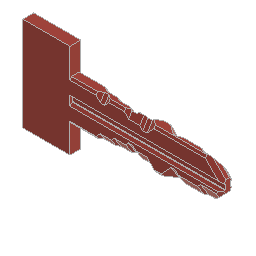
WR (Autodesk Fusion 360 design; units mm, degrees)
Autodesk Fusion 360 part; units mm, degrees
note: some values were not read from the file. Chosen so that the rebuilt part matches the saved one: which face or edge a step refers to. Set by a fixed rule: which sketch regions a step uses.
sketch "blade" plane through (0, 0, 0) normal (1, 0, 0) x (0, 1, 0)
  line L0 (0, 0) -> (1.15, 0) construction
  line L1 (1.15, 0) -> (1.15, 4.3)
  line L2 (1.15, 4.3) -> (-1.15, 4.3)
  line L3 (-1.15, 4.3) -> (-1.15, -4.3)
  line L4 (-1.15, -4.3) -> (1.15, -4.3)
  line L5 (1.15, -4.3) -> (1.15, 0)
  dimension "d61" = 1.15
  dimension "d62" = 4.3
  dimension "d63" = 2.3
  dimension "d64" = 8.6
  constraint coincident L0.start origin
  constraint horizontal L0
  constraint perpendicular L0 L1
  constraint perpendicular L1 L2
  constraint perpendicular L2 L3
  constraint perpendicular L1 L4
  constraint perpendicular L0 L5
  measures "d61" distance of L0.start L0.end
  measures "d62" distance of L0.end L1.end
  measures "d63" distance of L1.end L2.end
  measures "d64" distance of L2.end L3.end
extrude "Extrude1" add sketch "blade" against normal blind 32.35
sketch "centerline" plane through (0, 0, 0) normal (0, 0, 1) x (1, 0, 0)
  line L0 (0, 0) -> (-32.35, 0) construction
  dimension "d67" = 32.35
  constraint coincident L0.start origin
  constraint horizontal L0
  measures "d67" distance of L0.start L0.end
sketch "tip" plane through (0, 0, 0) normal (0, 1, 0) x (1, 0, 0)
  line L0 (0, 0) -> (0, -1.25) construction
  line L1 (0, -1.25) -> (-3.05, -4.3)
  line L2 (0, -1.25) -> (1.25, -1.25) construction
  line L3 (0, 0) -> (1.25, 0) construction
  line L4 (1.25, 0) -> (1.25, -1.25) construction
  line L5 (-3.05, -4.3) -> (0, -4.3)
  line L6 (0, -4.3) -> (0, -1.25)
  line L7 (0, 4.3) -> (0, 1.25)
  line L8 (0, 1.25) -> (-3.05, 4.3)
  line L9 (-3.05, 4.3) -> (0, 4.3)
  dimension "d68" = 1.25
  dimension "d69" = 135
  dimension "d70" = 4.3134
  dimension "d71" = 1.25
  dimension "d72" = 1.25
  constraint coincident L0.start L3.start
  constraint vertical L0
  constraint horizontal L2
  constraint perpendicular L0 L3
  constraint perpendicular L3 L4
  constraint perpendicular L0 L5
  constraint perpendicular L2 L6
  constraint symmetric L0.end L3 L7.end
  constraint symmetric L1.end L3 L8.end
  constraint symmetric L3 L5.end L7.start
  measures "d68" distance of L0.start L0.end
  measures "d69" angle of L1 L2
  measures "d70" distance of L0.end L1.end
  measures "d71" distance of L0.start L3.end
  measures "d72" distance of L3.end L2.end
sketch "warding" plane through (0, 0, 0) normal (1, 0, 0) x (0, 1, 0)
  line L0 (1.15, -4.3) -> (1.15, 4.3)
  line L1 (1.15, 4.3) -> (-1.15, 4.3)
  line L2 (-1.15, 4.3) -> (-1.15, -4.3)
  line L3 (-1.15, -4.3) -> (1.15, -4.3)
  line L4 (0, 0) -> (0.5, 0) construction
  line L5 (0.5, 0) -> (0.5, 0.5)
  line L6 (0.5, 0) -> (0.5, -0.5)
  line L7 (0.5, 0.5) -> (1.15, 0.5)
  line L8 (0.5, -0.5) -> (1.15, -0.5)
  line L9 (0, 0) -> (0, 0.5) construction
  line L10 (-0.5, -0.5) -> (-1.15, -0.5)
  line L11 (-0.5, 0) -> (-0.5, -0.5)
  line L12 (-0.5, 0) -> (-0.5, 0.5)
  line L13 (-0.5, 0.5) -> (-1.15, 0.5)
  dimension "d73" = 0.5
  dimension "d74" = 0.5
  dimension "d75" = 0.5
  dimension "d76" = 0.5
  constraint coincident L4.start L9.start
  constraint perpendicular L0 L4
  constraint perpendicular L4 L5
  constraint perpendicular L4 L6
  constraint coincident L0 L7.end
  constraint perpendicular L0 L7
  constraint coincident L0 L8.end
  constraint perpendicular L0 L8
  constraint perpendicular L4 L9
  constraint symmetric L4.end L9 L11.start
  constraint symmetric L5.end L9 L12.end
  constraint symmetric L6.end L9 L10.start
  constraint symmetric L7.end L9 L13.end
  constraint symmetric L8.end L9 L10.end
  measures "d73" distance of L4.start L4.end
  measures "d74" distance of L4.end L5.end
  measures "d75" distance of L4.end L6.end
  measures "d76" distance of L4.start L9.end
extrude "Extrude2" cut sketch "warding" against normal blind 32.35 contours L0 L5 L6 L7 L8 | L2 L10 L11 L12 L13
chamfer "Chamfer1" distance 0.5 angle 45 4 edges at (-16.175, -1.15, -0.5) (-16.175, 1.15, -0.5) (-16.175, -1.15, 0.5) (-16.175, 1.15, 0.5)
extrude "Extrude3" cut sketch "tip" along normal mid plane 2.3
chamfer "Chamfer2" distance 0.75 angle 45 4 edges at (-1.525, -1.15, 2.775) (-1.525, 1.15, 2.775) (-1.525, -1.15, -2.775) (-1.525, 1.15, -2.775)
ref_plane "WorkPlane1" through (-16.175, 0, 0) normal (0, 0.5373, 0.843391) x (-1, 0, 0)
ref_plane "WorkPlane2" through (-16.175, 0, 0) normal (0, -0.5373, 0.843391) x (-1, 0, 0)
sketch "tr_bl" plane through (0, 0, 0) normal (0, 0.5373, 0.843391) x (-1, 0, 0)
  line L0 (32.35, 0) -> (25.95, 0) construction
  line L1 (25.95, 0) -> (25.45, 0) construction
  line L2 (25.45, 0) -> (25.45, 2.5) construction
  line L3 (25.45, 0) -> (22.45, 0) construction
  line L4 (22.45, 0) -> (22.45, 3) construction
  line L5 (22.45, 0) -> (19.45, 0) construction
  line L6 (19.45, 0) -> (19.45, 2.5) construction
  line L7 (19.45, 0) -> (16.45, 0) construction
  line L8 (16.45, 0) -> (16.45, 2.15) construction
  line L9 (16.45, 0) -> (13.45, 0) construction
  line L10 (13.45, 0) -> (13.45, 3) construction
  line L11 (13.45, 0) -> (10.45, 0) construction
  line L12 (10.45, 0) -> (10.45, 3) construction
  line L13 (10.45, 0) -> (7.45, 0) construction
  line L14 (7.45, 0) -> (7.45, 3) construction
  line L15 (7.45, 0) -> (3.95, 0) construction
  line L16 (3.95, 0) -> (3.95, 3) construction
  line L17 (3.95, 3) -> (0, 3)
  line L18 (0, 3) -> (0, 0) construction
  line L19 (32.35, 0) -> (32.35, 3) construction
  line L20 (32.35, 3) -> (30.45, 3) construction
  line L21 (25.45, 2.5) -> (25.9108, 2.5)
  line L22 (25.45, 0) -> (28.45, 0) construction
  line L23 (28.45, 0) -> (28.45, 3) construction
  line L24 (30.45, 3) -> (28.45, 3)
  line L25 (28.45, 3) -> (26.7768, 3)
  line L26 (26.7768, 3) -> (25.9108, 2.5)
  line L27 (25.45, 2.5) -> (24.9892, 2.5)
  line L28 (22.45, 3) -> (24.1232, 3)
  line L29 (22.45, 3) -> (20.7768, 3)
  line L30 (19.45, 2.5) -> (19.9108, 2.5)
  line L31 (19.45, 2.5) -> (17.517, 2.5)
  line L32 (16.45, 2.15) -> (16.9108, 2.15)
  line L33 (16.45, 2.15) -> (15.9892, 2.15)
  line L34 (13.45, 3) -> (14.517, 3)
  line L35 (13.45, 3) -> (12.9892, 3)
  line L36 (10.45, 3) -> (10.9108, 3)
  line L37 (10.45, 3) -> (9.9892, 3)
  line L38 (7.45, 3) -> (7.9108, 3)
  line L39 (7.45, 3) -> (6.7392, 3)
  line L40 (3.95, 3) -> (4.6608, 3)
  line L41 (4.6608, 3) -> (6.7392, 3)
  line L42 (7.9108, 3) -> (9.9892, 3)
  line L43 (10.9108, 3) -> (12.9892, 3)
  line L44 (14.517, 3) -> (15.9892, 2.15)
  line L45 (16.9108, 2.15) -> (17.517, 2.5)
  line L46 (19.9108, 2.5) -> (20.7768, 3)
  line L47 (24.1232, 3) -> (24.9892, 2.5)
  line L48 (22.45, 0) -> (22.45, -3) construction
  line L49 (10.9108, -3) -> (12.9892, -3)
  line L50 (10.45, -3) -> (9.9892, -3)
  line L51 (25.45, -2.5) -> (25.9108, -2.5)
  line L52 (10.45, 0) -> (10.45, -3) construction
  line L53 (16.9108, -2.15) -> (17.517, -2.5)
  line L54 (25.45, -2.5) -> (24.9892, -2.5)
  line L55 (3.95, -3) -> (0, -3)
  line L56 (7.45, -3) -> (6.7392, -3)
  line L57 (26.7768, -3) -> (25.9108, -2.5)
  line L58 (32.35, -3) -> (30.45, -3) construction
  line L59 (10.45, -3) -> (10.9108, -3)
  line L60 (16.45, 0) -> (16.45, -2.15) construction
  line L61 (22.45, -3) -> (20.7768, -3)
  line L62 (24.1232, -3) -> (24.9892, -2.5)
  line L63 (19.45, 0) -> (19.45, -2.5) construction
  line L64 (28.45, 0) -> (28.45, -3) construction
  line L65 (7.45, -3) -> (7.9108, -3)
  line L66 (13.45, 0) -> (13.45, -3) construction
  line L67 (19.9108, -2.5) -> (20.7768, -3)
  line L68 (19.45, -2.5) -> (17.517, -2.5)
  line L69 (30.45, -3) -> (28.45, -3)
  line L70 (28.45, -3) -> (26.7768, -3)
  line L71 (22.45, -3) -> (24.1232, -3)
  line L72 (16.45, -2.15) -> (16.9108, -2.15)
  line L73 (19.45, -2.5) -> (19.9108, -2.5)
  line L74 (13.45, -3) -> (14.517, -3)
  line L75 (25.45, 0) -> (25.45, -2.5) construction
  line L76 (32.35, 0) -> (32.35, -3) construction
  line L77 (7.45, 0) -> (7.45, -3) construction
  line L78 (13.45, -3) -> (12.9892, -3)
  line L79 (3.95, 0) -> (3.95, -3) construction
  line L80 (3.95, -3) -> (4.6608, -3)
  line L81 (0, -3) -> (0, 0) construction
  line L82 (14.517, -3) -> (15.9892, -2.15)
  line L83 (16.45, -2.15) -> (15.9892, -2.15)
  line L84 (7.9108, -3) -> (9.9892, -3)
  line L85 (4.6608, -3) -> (6.7392, -3)
  point P0 (32.35, 0)
  point P1 (32.35, 0)
  dimension "d86" = 6.4
  dimension "d87" = 0.5
  dimension "d88" = 2.5
  dimension "d89" = 3
  dimension "d90" = 3
  dimension "d91" = 3
  dimension "d92" = 2.5
  dimension "d93" = 3
  dimension "d94" = 2.15
  dimension "d95" = 3
  dimension "d96" = 3
  dimension "d97" = 3
  dimension "d98" = 3
  dimension "d99" = 3
  dimension "d100" = 3
  dimension "d101" = 3.5
  dimension "d102" = 3
  dimension "d103" = 3
  dimension "d104" = 1.9
  dimension "d105" = 0.4608
  dimension "d106" = 3
  dimension "d107" = 3
  dimension "d108" = 1.6732
  dimension "d109" = 0.4608
  dimension "d110" = 1.6732
  dimension "d111" = 1.6732
  dimension "d112" = 0.4608
  dimension "d113" = 1.933
  dimension "d114" = 0.4608
  dimension "d115" = 0.4608
  dimension "d116" = 1.067
  dimension "d117" = 0.4608
  dimension "d118" = 0.4608
  dimension "d119" = 0.4608
  dimension "d120" = 0.4608
  dimension "d121" = 0.7108
  dimension "d122" = 0.7108
  constraint coincident P0 L0.start
  constraint coincident P1 P0
  constraint horizontal L0
  constraint parallel L0 L1
  constraint perpendicular L1 L2
  constraint perpendicular L2 L3
  constraint perpendicular L3 L4
  constraint perpendicular L4 L5
  constraint perpendicular L5 L6
  constraint perpendicular L6 L7
  constraint perpendicular L7 L8
  constraint perpendicular L8 L9
  constraint perpendicular L9 L10
  constraint perpendicular L10 L11
  constraint perpendicular L11 L12
  constraint perpendicular L12 L13
  constraint perpendicular L13 L14
  constraint perpendicular L14 L15
  constraint perpendicular L15 L16
  constraint perpendicular L16 L17
  constraint coincident L18.end L81.end
  constraint perpendicular L17 L18
  constraint perpendicular L0 L19
  constraint perpendicular L19 L20
  constraint perpendicular L2 L21
  constraint perpendicular L2 L22
  constraint perpendicular L22 L23
  constraint perpendicular L23 L25
  constraint perpendicular L2 L27
  constraint perpendicular L4 L28
  constraint perpendicular L4 L29
  constraint perpendicular L6 L30
  constraint perpendicular L6 L31
  constraint perpendicular L8 L32
  constraint perpendicular L8 L33
  constraint perpendicular L10 L34
  constraint perpendicular L10 L35
  constraint perpendicular L12 L36
  constraint perpendicular L12 L37
  constraint perpendicular L14 L38
  constraint perpendicular L14 L39
  constraint perpendicular L16 L40
  constraint symmetric L1.end L7 L2.start
  constraint symmetric L2.end L7 L51.start
  constraint symmetric L3.end L7 L4.start
  constraint symmetric L4.end L7 L48.end
  constraint symmetric L5.end L7 L6.start
  constraint symmetric L6.end L7 L63.end
  constraint symmetric L8.start L7 L9.start
  constraint symmetric L7 L8.end L60.end
  constraint symmetric L7 L9.end L10.start
  constraint symmetric L7 L10.end L66.end
  constraint symmetric L7 L11.end L12.start
  constraint symmetric L7 L12.end L50.start
  constraint symmetric L7 L13.end L14.start
  constraint symmetric L7 L14.end L56.start
  constraint symmetric L7 L15.end L16.start
  constraint symmetric L7 L16.end L55.start
  constraint symmetric L7 L17.end L55.end
  constraint symmetric L7 L18.end L81.end
  constraint symmetric L7 P1 P0
  constraint symmetric L7 L19.end L58.start
  constraint symmetric L7 L20.end L58.end
  constraint symmetric L7 L21.end L51.end
  constraint symmetric L7 L22.end L23.start
  constraint symmetric L7 L23.end L64.end
  constraint symmetric L7 L25.end L57.start
  constraint symmetric L7 L27.end L54.end
  constraint symmetric L7 L28.end L62.start
  constraint symmetric L7 L29.end L61.end
  constraint symmetric L7 L30.end L67.start
  constraint symmetric L7 L31.end L53.end
  constraint symmetric L7 L32.end L53.start
  constraint symmetric L7 L33.end L82.end
  constraint symmetric L7 L34.end L74.end
  constraint symmetric L7 L35.end L49.end
  constraint symmetric L7 L36.end L49.start
  constraint symmetric L7 L37.end L50.end
  constraint symmetric L7 L38.end L65.end
  constraint symmetric L7 L39.end L56.end
  constraint symmetric L7 L40.end L80.end
  measures "d86" distance of P1 L0.end
  measures "d87" distance of L0.end L1.end
  measures "d88" distance of L1.end L2.end
  measures "d89" distance of L1.end L3.end
  measures "d90" distance of L3.end L4.end
  measures "d91" distance of L3.end L5.end
  measures "d92" distance of L5.end L6.end
  measures "d93" distance of L5.end L7.end
  measures "d94" distance of L7.end L8.end
  measures "d95" distance of L7.end L9.end
  measures "d96" distance of L9.end L10.end
  measures "d97" distance of L9.end L11.end
  measures "d98" distance of L11.end L12.end
  measures "d99" distance of L11.end L13.end
  measures "d100" distance of L13.end L14.end
  measures "d101" distance of L13.end L15.end
  measures "d102" distance of L15.end L16.end
  measures "d103" distance of P1 L19.end
  measures "d104" distance of L19.end L20.end
  measures "d105" distance of L2.end L21.end
  measures "d106" distance of L1.end L22.end
  measures "d107" distance of L22.end L23.end
  measures "d108" distance of L23.end L25.end
  measures "d109" distance of L2.end L27.end
  measures "d110" distance of L4.end L28.end
  measures "d111" distance of L4.end L29.end
  measures "d112" distance of L6.end L30.end
  measures "d113" distance of L6.end L31.end
  measures "d114" distance of L8.end L32.end
  measures "d115" distance of L8.end L33.end
  measures "d116" distance of L10.end L34.end
  measures "d117" distance of L10.end L35.end
  measures "d118" distance of L12.end L36.end
  measures "d119" distance of L12.end L37.end
  measures "d120" distance of L14.end L38.end
  measures "d121" distance of L14.end L39.end
  measures "d122" distance of L16.end L40.end
sketch "tr_bl cutters" plane through (0, 0, 0) normal (1, 0, 0) x (0, 1, 0)
  line L0 (0, 0) -> (-2.5302, 1.6119) construction
  line L1 (0, 0) -> (-3.5571, 0) construction
  line L2 (-2.5302, 1.6119) -> (-0.1123, 5.4072)
  line L3 (-2.5302, 1.6119) -> (-4.948, -2.1834)
  line L4 (-0.1123, 5.4072) -> (-4.948, 5.4072)
  line L5 (-4.948, 5.4072) -> (-4.948, -2.1834)
  line L6 (0, 0) -> (2.5302, -1.6119) construction
  line L7 (2.5302, -1.6119) -> (0.1123, -5.4072)
  line L8 (2.5302, -1.6119) -> (4.948, 2.1834)
  line L9 (0.1123, -5.4072) -> (4.948, -5.4072)
  line L10 (4.948, -5.4072) -> (4.948, 2.1834)
  dimension "d123" = 147.5
  dimension "d124" = 3
  dimension "d126" = 4.5
  dimension "d127" = 4.5
  dimension "d128" = 3
  dimension "d129" = 4.5
  dimension "d130" = 4.5
  constraint horizontal L1
  constraint coincident L0.start L1.start
  constraint perpendicular L0 L2
  constraint perpendicular L0 L3
  constraint horizontal L4
  constraint perpendicular L4 L5
  constraint coincident L1.end L3
  constraint parallel L0 L6
  constraint perpendicular L6 L7
  constraint perpendicular L6 L8
  constraint horizontal L9
  constraint perpendicular L9 L10
  measures "d123" angle of L0 L1
  measures "d124" distance of L0.start L0.end
  measures "d126" distance of L0.end L2.end
  measures "d127" distance of L0.end L3.end
  measures "d128" distance of L0.start L6.end
  measures "d129" distance of L6.end L7.end
  measures "d130" distance of L6.end L8.end
sketch "tl_br" plane through (0, 0, 0) normal (0, -0.5373, 0.843391) x (-1, 0, 0)
  line L0 (32.35, 0) -> (25.95, 0) construction
  line L1 (25.95, 0) -> (25.45, 0) construction
  line L2 (25.45, 0) -> (25.45, -2.5) construction
  line L3 (25.45, 0) -> (22.45, 0) construction
  line L4 (22.45, 0) -> (22.45, -2.15) construction
  line L5 (22.45, 0) -> (19.45, 0) construction
  line L6 (19.45, 0) -> (19.45, -1.8) construction
  line L7 (19.45, 0) -> (16.45, 0) construction
  line L8 (16.45, 0) -> (16.45, -2.15) construction
  line L9 (16.45, 0) -> (13.45, 0) construction
  line L10 (13.45, 0) -> (13.45, -3) construction
  line L11 (13.45, 0) -> (10.45, 0) construction
  line L12 (10.45, 0) -> (10.45, -1.8) construction
  line L13 (10.45, 0) -> (7.45, 0) construction
  line L14 (7.45, 0) -> (7.45, -2.15) construction
  line L15 (7.45, 0) -> (3.95, 0) construction
  line L16 (3.95, 0) -> (3.95, -1.8) construction
  line L17 (3.95, -1.8) -> (0, -1.8)
  line L18 (0, -1.8) -> (0, 0) construction
  line L19 (32.35, 0) -> (32.35, -3) construction
  line L20 (32.35, -3) -> (30.45, -3) construction
  line L21 (25.45, 0) -> (28.45, 0) construction
  line L22 (28.45, 0) -> (28.45, -3) construction
  line L23 (28.45, -3) -> (30.45, -3)
  line L24 (25.45, -2.5) -> (25.9108, -2.5)
  line L25 (28.45, -3) -> (26.7768, -3)
  line L26 (26.7768, -3) -> (25.9108, -2.5)
  line L27 (25.45, -2.5) -> (23.517, -2.5)
  line L28 (22.45, -2.15) -> (22.9108, -2.15)
  line L29 (22.45, -2.15) -> (20.517, -2.15)
  line L30 (19.45, -1.8) -> (19.9108, -1.8)
  line L31 (19.45, -1.8) -> (18.9892, -1.8)
  line L32 (16.45, -2.15) -> (18.383, -2.15)
  line L33 (16.45, -2.15) -> (15.9892, -2.15)
  line L34 (13.45, -3) -> (14.517, -3)
  line L35 (13.45, -3) -> (12.9892, -3)
  line L36 (10.45, -1.8) -> (10.9108, -1.8)
  line L37 (10.45, -1.8) -> (9.9892, -1.8)
  line L38 (7.45, -2.15) -> (9.383, -2.15)
  line L39 (7.45, -2.15) -> (5.267, -2.15)
  line L40 (3.95, -1.8) -> (4.6608, -1.8)
  line L41 (4.6608, -1.8) -> (5.267, -2.15)
  line L42 (9.383, -2.15) -> (9.9892, -1.8)
  line L43 (10.9108, -1.8) -> (12.9892, -3)
  line L44 (14.517, -3) -> (15.9892, -2.15)
  line L45 (18.383, -2.15) -> (18.9892, -1.8)
  line L46 (19.9108, -1.8) -> (20.517, -2.15)
  line L47 (22.9108, -2.15) -> (23.517, -2.5)
  line L48 (22.45, 0) -> (22.45, 2.15) construction
  line L49 (19.45, 1.8) -> (18.9892, 1.8)
  line L50 (22.45, 2.15) -> (20.517, 2.15)
  line L51 (22.45, 2.15) -> (22.9108, 2.15)
  line L52 (19.9108, 1.8) -> (20.517, 2.15)
  line L53 (25.45, 2.5) -> (23.517, 2.5)
  line L54 (7.45, 2.15) -> (9.383, 2.15)
  line L55 (7.45, 0) -> (7.45, 2.15) construction
  line L56 (3.95, 0) -> (3.95, 1.8) construction
  line L57 (28.45, 3) -> (30.45, 3)
  line L58 (28.45, 0) -> (28.45, 3) construction
  line L59 (25.45, 0) -> (25.45, 2.5) construction
  line L60 (0, 1.8) -> (0, 0) construction
  line L61 (28.45, 3) -> (26.7768, 3)
  line L62 (32.35, 3) -> (30.45, 3) construction
  line L63 (25.45, 2.5) -> (25.9108, 2.5)
  line L64 (22.9108, 2.15) -> (23.517, 2.5)
  line L65 (9.383, 2.15) -> (9.9892, 1.8)
  line L66 (18.383, 2.15) -> (18.9892, 1.8)
  line L67 (19.45, 1.8) -> (19.9108, 1.8)
  line L68 (10.45, 1.8) -> (10.9108, 1.8)
  line L69 (16.45, 2.15) -> (18.383, 2.15)
  line L70 (10.45, 1.8) -> (9.9892, 1.8)
  line L71 (14.517, 3) -> (15.9892, 2.15)
  line L72 (10.9108, 1.8) -> (12.9892, 3)
  line L73 (13.45, 3) -> (14.517, 3)
  line L74 (13.45, 0) -> (13.45, 3) construction
  line L75 (13.45, 3) -> (12.9892, 3)
  line L76 (7.45, 2.15) -> (5.267, 2.15)
  line L77 (10.45, 0) -> (10.45, 1.8) construction
  line L78 (19.45, 0) -> (19.45, 1.8) construction
  line L79 (26.7768, 3) -> (25.9108, 2.5)
  line L80 (32.35, 0) -> (32.35, 3) construction
  line L81 (16.45, 2.15) -> (15.9892, 2.15)
  line L82 (3.95, 1.8) -> (4.6608, 1.8)
  line L83 (3.95, 1.8) -> (0, 1.8)
  line L84 (16.45, 0) -> (16.45, 2.15) construction
  line L85 (4.6608, 1.8) -> (5.267, 2.15)
  point P0 (32.35, 0)
  point P1 (32.35, 0)
  dimension "d131" = 6.4
  dimension "d132" = 0.5
  dimension "d133" = 2.5
  dimension "d134" = 3
  dimension "d135" = 2.15
  dimension "d136" = 3
  dimension "d137" = 1.8
  dimension "d138" = 3
  dimension "d139" = 2.15
  dimension "d140" = 3
  dimension "d141" = 3
  dimension "d142" = 3
  dimension "d143" = 1.8
  dimension "d144" = 3
  dimension "d145" = 2.15
  dimension "d146" = 3.5
  dimension "d147" = 1.8
  dimension "d148" = 3
  dimension "d149" = 1.9
  dimension "d150" = 3
  dimension "d151" = 3
  dimension "d152" = 0.4608
  dimension "d153" = 1.6732
  dimension "d154" = 1.933
  dimension "d155" = 0.4608
  dimension "d156" = 1.933
  dimension "d157" = 0.4608
  dimension "d158" = 0.4608
  dimension "d159" = 1.933
  dimension "d160" = 0.4608
  dimension "d161" = 1.067
  dimension "d162" = 0.4608
  dimension "d163" = 0.4608
  dimension "d164" = 0.4608
  dimension "d165" = 1.933
  dimension "d166" = 2.183
  dimension "d167" = 0.7108
  constraint coincident P0 L0.start
  constraint horizontal L0
  constraint parallel L0 L1
  constraint perpendicular L1 L2
  constraint perpendicular L2 L3
  constraint perpendicular L3 L4
  constraint perpendicular L4 L5
  constraint perpendicular L5 L6
  constraint perpendicular L6 L7
  constraint perpendicular L7 L8
  constraint perpendicular L8 L9
  constraint perpendicular L9 L10
  constraint perpendicular L10 L11
  constraint perpendicular L11 L12
  constraint perpendicular L12 L13
  constraint perpendicular L13 L14
  constraint perpendicular L14 L15
  constraint perpendicular L15 L16
  constraint perpendicular L16 L17
  constraint coincident L18.end L60.end
  constraint perpendicular L17 L18
  constraint coincident P1 P0
  constraint perpendicular L0 L19
  constraint perpendicular L19 L20
  constraint perpendicular L2 L21
  constraint perpendicular L21 L22
  constraint perpendicular L2 L24
  constraint perpendicular L22 L25
  constraint perpendicular L2 L27
  constraint perpendicular L4 L28
  constraint perpendicular L4 L29
  constraint perpendicular L6 L30
  constraint perpendicular L6 L31
  constraint perpendicular L8 L32
  constraint perpendicular L8 L33
  constraint perpendicular L10 L34
  constraint perpendicular L10 L35
  constraint perpendicular L12 L36
  constraint perpendicular L12 L37
  constraint perpendicular L14 L38
  constraint perpendicular L14 L39
  constraint perpendicular L16 L40
  constraint symmetric L1.end L7 L2.start
  constraint symmetric L2.end L7 L53.start
  constraint symmetric L3.end L7 L4.start
  constraint symmetric L4.end L7 L48.end
  constraint symmetric L5.end L7 L6.start
  constraint symmetric L6.end L7 L49.start
  constraint symmetric L8.start L7 L9.start
  constraint symmetric L7 L8.end L69.start
  constraint symmetric L7 L9.end L10.start
  constraint symmetric L7 L10.end L73.start
  constraint symmetric L7 L11.end L12.start
  constraint symmetric L7 L12.end L68.start
  constraint symmetric L7 L13.end L14.start
  constraint symmetric L7 L14.end L54.start
  constraint symmetric L7 L15.end L16.start
  constraint symmetric L7 L16.end L56.end
  constraint symmetric L7 L17.end L60.start
  constraint symmetric L7 L18.end L60.end
  constraint symmetric L7 P1 P0
  constraint symmetric L7 L19.end L62.start
  constraint symmetric L7 L20.end L57.end
  constraint symmetric L7 L21.end L22.start
  constraint symmetric L7 L22.end L57.start
  constraint symmetric L7 L24.end L63.end
  constraint symmetric L7 L25.end L61.end
  constraint symmetric L7 L27.end L53.end
  constraint symmetric L7 L28.end L51.end
  constraint symmetric L7 L29.end L50.end
  constraint symmetric L7 L30.end L52.start
  constraint symmetric L7 L31.end L49.end
  constraint symmetric L7 L32.end L66.start
  constraint symmetric L7 L33.end L71.end
  constraint symmetric L7 L34.end L71.start
  constraint symmetric L7 L35.end L72.end
  constraint symmetric L7 L36.end L68.end
  constraint symmetric L7 L37.end L65.end
  constraint symmetric L7 L38.end L54.end
  constraint symmetric L7 L39.end L76.end
  constraint symmetric L7 L40.end L82.end
  measures "d131" distance of P1 L0.end
  measures "d132" distance of L0.end L1.end
  measures "d133" distance of L1.end L2.end
  measures "d134" distance of L1.end L3.end
  measures "d135" distance of L3.end L4.end
  measures "d136" distance of L3.end L5.end
  measures "d137" distance of L5.end L6.end
  measures "d138" distance of L5.end L7.end
  measures "d139" distance of L7.end L8.end
  measures "d140" distance of L7.end L9.end
  measures "d141" distance of L9.end L10.end
  measures "d142" distance of L9.end L11.end
  measures "d143" distance of L11.end L12.end
  measures "d144" distance of L11.end L13.end
  measures "d145" distance of L13.end L14.end
  measures "d146" distance of L13.end L15.end
  measures "d147" distance of L15.end L16.end
  measures "d148" distance of P1 L19.end
  measures "d149" distance of L19.end L20.end
  measures "d150" distance of L1.end L21.end
  measures "d151" distance of L21.end L22.end
  measures "d152" distance of L2.end L24.end
  measures "d153" distance of L22.end L25.end
  measures "d154" distance of L2.end L27.end
  measures "d155" distance of L4.end L28.end
  measures "d156" distance of L4.end L29.end
  measures "d157" distance of L6.end L30.end
  measures "d158" distance of L6.end L31.end
  measures "d159" distance of L8.end L32.end
  measures "d160" distance of L8.end L33.end
  measures "d161" distance of L10.end L34.end
  measures "d162" distance of L10.end L35.end
  measures "d163" distance of L12.end L36.end
  measures "d164" distance of L12.end L37.end
  measures "d165" distance of L14.end L38.end
  measures "d166" distance of L14.end L39.end
  measures "d167" distance of L16.end L40.end
sketch "tl_br cutters" plane through (0, 0, 0) normal (1, 0, 0) x (0, 1, 0)
  line L0 (0, 0) -> (1.5181, 0.9671) construction
  line L1 (0, 0) -> (2.1342, 0) construction
  line L2 (1.5181, 0.9671) -> (-0.8997, 4.7624)
  line L3 (1.5181, 0.9671) -> (3.936, -2.8281)
  line L4 (-0.8997, 4.7624) -> (3.936, 4.7624)
  line L5 (3.936, 4.7624) -> (3.936, -2.8281)
  line L6 (0, 0) -> (-1.5181, -0.9671) construction
  line L7 (-1.5181, -0.9671) -> (-3.936, 2.8281)
  line L8 (-1.5181, -0.9671) -> (0.8997, -4.7624)
  line L9 (0.8997, -4.7624) -> (-3.936, -4.7624)
  line L10 (-3.936, -4.7624) -> (-3.936, 2.8281)
  dimension "d168" = 1.8
  dimension "d169" = 32.5
  dimension "d170" = 4.5
  dimension "d171" = 4.5
  dimension "d172" = 1.8
  dimension "d173" = 4.5
  dimension "d174" = 4.5
  constraint horizontal L1
  constraint coincident L0.start L1.start
  constraint perpendicular L0 L2
  constraint perpendicular L0 L3
  constraint coincident L1.end L3
  constraint horizontal L4
  constraint perpendicular L4 L5
  constraint parallel L0 L6
  constraint perpendicular L6 L7
  constraint perpendicular L6 L8
  constraint horizontal L9
  constraint perpendicular L9 L10
  measures "d168" distance of L0.start L0.end
  measures "d169" angle of L0 L1
  measures "d170" distance of L0.end L2.end
  measures "d171" distance of L0.end L3.end
  measures "d172" distance of L0.start L6.end
  measures "d173" distance of L6.end L7.end
  measures "d174" distance of L6.end L8.end
sweep "Sweep1" cut profiles "tr_bl cutters" path "tr_bl" along L17 L40 L41 L39 L38 L42 L37 L36 L43 L35 L34 L44 L33 L32 L45 L31 L30 L46 L29 L28 L47 L27 L21 L26 L25 L24 section 1 contours L2 L3 L4 L5
sweep "Sweep2" cut profiles "tr_bl cutters" path "tr_bl" along L69 L70 L57 L51 L54 L62 L71 L61 L67 L73 L68 L53 L72 L83 L82 L74 L78 L49 L59 L50 L84 L65 L56 L85 L80 L55 section 1 contours L7 L8 L9 L10
sweep "Sweep3" cut profiles "tl_br cutters" path "tl_br" along L23 L25 L26 L24 L27 L47 L28 L29 L46 L30 L31 L45 L32 L33 L44 L34 L35 L43 L36 L37 L42 L38 L39 L41 L40 L17 section 1 contours L2 L3 L4 L5
sweep "Sweep4" cut profiles "tl_br cutters" path "tl_br" along L83 L82 L85 L76 L54 L65 L70 L68 L72 L75 L73 L71 L81 L69 L66 L49 L67 L52 L50 L51 L64 L53 L63 L79 L61 L57 section 1 contours L7 L8 L9 L10
sketch "Sketch9" plane through (-32.35, 0, 0) normal (-1, 0, 0) x (0, -1, 0)
  line L0 (-1.15, 1) -> (-0.65, 0.5)
  line L1 (-0.65, 0.5) -> (-0.5, 0.5)
  line L2 (-0.5, 0.5) -> (-0.5, -0.5)
  line L3 (-0.5, -0.5) -> (-0.65, -0.5)
  line L4 (-0.65, -0.5) -> (-1.15, -1)
  line L5 (-1.15, -1) -> (-1.15, -4.3)
  line L6 (-1.15, -4.3) -> (1.15, -4.3)
  line L7 (1.15, -4.3) -> (1.15, -1)
  line L8 (1.15, -1) -> (0.65, -0.5)
  line L9 (0.65, -0.5) -> (0.5, -0.5)
  line L10 (0.5, -0.5) -> (0.5, 0.5)
  line L11 (0.5, 0.5) -> (0.65, 0.5)
  line L12 (0.65, 0.5) -> (1.15, 1)
  line L13 (1.15, 1) -> (1.15, 4.3)
  line L14 (1.15, 4.3) -> (-1.15, 4.3)
  line L15 (-1.15, 4.3) -> (-1.15, 1)
  line L16 (1.15, 10) -> (-1.15, 10)
  line L17 (-1.15, 10) -> (-1.15, -10)
  line L18 (-1.15, -10) -> (1.15, -10)
  line L19 (1.15, -10) -> (1.15, 10)
  line L20 (1.15, 10) -> (-1.15, -10) construction
  line L21 (-1.15, 10) -> (1.15, -10) construction
  dimension "d199" = 2.3
  dimension "d200" = 20
  constraint horizontal L16
  constraint perpendicular L16 L17
  constraint parallel L16 L18
  constraint parallel L17 L19
  constraint coincident L20 origin
  constraint coincident L21 origin
  measures "d199" distance of L17.end L18.end
  measures "d200" distance of L16.end L17.end
extrude "Extrude4" add sketch "Sketch9" along normal blind 10
extrude "Extrude5" cut 4 faces at (-30.45, 1.0392, 4.1261) (-30.45, -1.0392, 4.1261) (-30.45, 1.0392, -4.1261) (-30.45, -1.0392, -4.1261) along direction (-1, 0, 0) blind 1.9
equation "tr_bl1 = 1"
equation "trbl1 = ( -0.025 * tr_bl1 ^ 3 + 0.15 * tr_bl1 ^ 2 - 0.625 * tr_bl1 + 3 )"
equation "tr_bl2 = 0"
equation "trbl2 = ( -0.025 * tr_bl2 ^ 3 + 0.15 * tr_bl2 ^ 2 - 0.625 * tr_bl2 + 3 )"
equation "tr_bl3 = 1"
equation "trbl3 = ( -0.025 * tr_bl3 ^ 3 + 0.15 * tr_bl3 ^ 2 - 0.625 * tr_bl3 + 3 )"
equation "tr_bl4 = 2"
equation "trbl4 = ( -0.025 * tr_bl4 ^ 3 + 0.15 * tr_bl4 ^ 2 - 0.625 * tr_bl4 + 3 )"
equation "tr_bl5 = 0"
equation "trbl5 = ( -0.025 * tr_bl5 ^ 3 + 0.15 * tr_bl5 ^ 2 - 0.625 * tr_bl5 + 3 )"
equation "tr_bl6 = 0"
equation "trbl6 = ( -0.025 * tr_bl6 ^ 3 + 0.15 * tr_bl6 ^ 2 - 0.625 * tr_bl6 + 3 )"
equation "tr_bl7 = 0"
equation "trbl7 = ( -0.025 * tr_bl7 ^ 3 + 0.15 * tr_bl7 ^ 2 - 0.625 * tr_bl7 + 3 )"
equation "tr_bl8 = 0"
equation "trbl8 = ( -0.025 * tr_bl8 ^ 3 + 0.15 * tr_bl8 ^ 2 - 0.625 * tr_bl8 + 3 )"
equation "tr1_right = if(( trbl1 > trbl2 ) and ( ( abs(trbl1 - trbl2) ) <> 1.2 ) and ( ( trbl1 - trbl2 ) <> 0 ); 3 mm - ( ( 3 mm - ( ( ( 2.4 * cos(30 deg) ) * 1 mm ) ) ) / 2 ) - ( ( ( trbl1 - trbl2 ) * 2 * cos(30 deg) ) * 1 mm ); if(( trbl1 < trbl2 ) and ( ( abs(trbl1 - trbl2) ) <> 1.2 ) and ( ( trbl1 - trbl2 ) <> 0 ); ( ( 3 - ( 2.40 * cos(30 deg) ) ) / 2 ) * 1 mm; if(( ( abs(trbl1 - trbl2) ) <> 1.2 ) or ( ( trbl1 - trbl2 ) <> 0 ); ( ( 3 - ( 2.40 * cos(30 deg) ) ) / 2 ) * 1 mm; 1 mm)))"
equation "tr2_left = if(( trbl1 < trbl2 ) and ( ( abs(trbl1 - trbl2) ) <> 1.2 ) and ( ( trbl1 - trbl2 ) <> 0 ); 3 mm - ( ( 3 mm - ( ( ( 2.4 * cos(30 deg) ) * 1 mm ) ) ) / 2 ) - ( ( ( trbl2 - trbl1 ) * 2 * cos(30 deg) ) * 1 mm ); if(( trbl1 > trbl2 ) and ( ( abs(trbl1 - trbl2) ) <> 1.2 ) and ( ( trbl1 - trbl2 ) <> 0 ); ( ( 3 - ( 2.40 * cos(30 deg) ) ) / 2 ) * 1 mm; if(( ( abs(trbl2 - trbl1) ) <> 1.2 ) or ( ( trbl1 - trbl2 ) <> 0 ); ( ( 3 - ( 2.40 * cos(30 deg) ) ) / 2 ) * 1 mm; 1 mm)))"
equation "tr2_right = if(( trbl2 > trbl3 ) and ( ( abs(trbl2 - trbl3) ) <> 1.2 ) and ( ( trbl2 - trbl3 ) <> 0 ); 3 mm - ( ( 3 mm - ( ( ( 2.4 * cos(30 deg) ) * 1 mm ) ) ) / 2 ) - ( ( ( trbl2 - trbl3 ) * 2 * cos(30 deg) ) * 1 mm ); if(( trbl2 < trbl3 ) and ( ( abs(trbl2 - trbl3) ) <> 1.2 ) and ( ( trbl2 - trbl3 ) <> 0 ); ( ( 3 - ( 2.40 * cos(30 deg) ) ) / 2 ) * 1 mm; if(( ( abs(trbl2 - trbl3) ) <> 1.2 ) or ( ( trbl2 - trbl3 ) <> 0 ); ( ( 3 - ( 2.40 * cos(30 deg) ) ) / 2 ) * 1 mm; 1 mm)))"
equation "tr3_left = if(( trbl2 < trbl3 ) and ( ( abs(trbl2 - trbl3) ) <> 1.2 ) and ( ( trbl2 - trbl3 ) <> 0 ); 3 mm - ( ( 3 mm - ( ( ( 2.4 * cos(30 deg) ) * 1 mm ) ) ) / 2 ) - ( ( ( trbl3 - trbl2 ) * 2 * cos(30 deg) ) * 1 mm ); if(( trbl2 > trbl3 ) and ( ( abs(trbl2 - trbl3) ) <> 1.2 ) and ( ( trbl2 - trbl3 ) <> 0 ); ( ( 3 - ( 2.40 * cos(30 deg) ) ) / 2 ) * 1 mm; if(( ( abs(trbl3 - trbl2) ) <> 1.2 ) or ( ( trbl2 - trbl3 ) <> 0 ); ( ( 3 - ( 2.40 * cos(30 deg) ) ) / 2 ) * 1 mm; 1 mm)))"
equation "tr3_right = if(( trbl3 > trbl4 ) and ( ( abs(trbl3 - trbl4) ) <> 1.2 ) and ( ( trbl3 - trbl4 ) <> 0 ); 3 mm - ( ( 3 mm - ( ( ( 2.4 * cos(30 deg) ) * 1 mm ) ) ) / 2 ) - ( ( ( trbl3 - trbl4 ) * 2 * cos(30 deg) ) * 1 mm ); if(( trbl3 < trbl4 ) and ( ( abs(trbl3 - trbl4) ) <> 1.2 ) and ( ( trbl3 - trbl4 ) <> 0 ); ( ( 3 - ( 2.40 * cos(30 deg) ) ) / 2 ) * 1 mm; if(( ( abs(trbl3 - trbl4) ) <> 1.2 ) or ( ( trbl3 - trbl4 ) <> 0 ); ( ( 3 - ( 2.40 * cos(30 deg) ) ) / 2 ) * 1 mm; 1 mm)))"
equation "tr4_left = if(( trbl3 < trbl4 ) and ( ( abs(trbl3 - trbl4) ) <> 1.2 ) and ( ( trbl3 - trbl4 ) <> 0 ); 3 mm - ( ( 3 mm - ( ( ( 2.4 * cos(30 deg) ) * 1 mm ) ) ) / 2 ) - ( ( ( trbl4 - trbl3 ) * 2 * cos(30 deg) ) * 1 mm ); if(( trbl3 > trbl4 ) and ( ( abs(trbl3 - trbl4) ) <> 1.2 ) and ( ( trbl3 - trbl4 ) <> 0 ); ( ( 3 - ( 2.40 * cos(30 deg) ) ) / 2 ) * 1 mm; if(( ( abs(trbl4 - trbl3) ) <> 1.2 ) or ( ( trbl3 - trbl4 ) <> 0 ); ( ( 3 - ( 2.40 * cos(30 deg) ) ) / 2 ) * 1 mm; 1 mm)))"
equation "tr4_right = if(( trbl4 > trbl5 ) and ( ( abs(trbl4 - trbl5) ) <> 1.2 ) and ( ( trbl4 - trbl5 ) <> 0 ); 3 mm - ( ( 3 mm - ( ( ( 2.4 * cos(30 deg) ) * 1 mm ) ) ) / 2 ) - ( ( ( trbl4 - trbl5 ) * 2 * cos(30 deg) ) * 1 mm ); if(( trbl4 < trbl5 ) and ( ( abs(trbl4 - trbl5) ) <> 1.2 ) and ( ( trbl4 - trbl5 ) <> 0 ); ( ( 3 - ( 2.40 * cos(30 deg) ) ) / 2 ) * 1 mm; if(( ( abs(trbl4 - trbl5) ) <> 1.2 ) or ( ( trbl4 - trbl5 ) <> 0 ); ( ( 3 - ( 2.40 * cos(30 deg) ) ) / 2 ) * 1 mm; 1 mm)))"
equation "tr5_left = if(( trbl4 < trbl5 ) and ( ( abs(trbl4 - trbl5) ) <> 1.2 ) and ( ( trbl4 - trbl5 ) <> 0 ); 3 mm - ( ( 3 mm - ( ( ( 2.4 * cos(30 deg) ) * 1 mm ) ) ) / 2 ) - ( ( ( trbl5 - trbl4 ) * 2 * cos(30 deg) ) * 1 mm ); if(( trbl4 > trbl5 ) and ( ( abs(trbl4 - trbl5) ) <> 1.2 ) and ( ( trbl4 - trbl5 ) <> 0 ); ( ( 3 - ( 2.40 * cos(30 deg) ) ) / 2 ) * 1 mm; if(( ( abs(trbl5 - trbl4) ) <> 1.2 ) or ( ( trbl4 - trbl5 ) <> 0 ); ( ( 3 - ( 2.40 * cos(30 deg) ) ) / 2 ) * 1 mm; 1 mm)))"
equation "tr5_right = if(( trbl5 > trbl6 ) and ( ( abs(trbl5 - trbl6) ) <> 1.2 ) and ( ( trbl5 - trbl6 ) <> 0 ); 3 mm - ( ( 3 mm - ( ( ( 2.4 * cos(30 deg) ) * 1 mm ) ) ) / 2 ) - ( ( ( trbl5 - trbl6 ) * 2 * cos(30 deg) ) * 1 mm ); if(( trbl5 < trbl6 ) and ( ( abs(trbl5 - trbl6) ) <> 1.2 ) and ( ( trbl5 - trbl6 ) <> 0 ); ( ( 3 - ( 2.40 * cos(30 deg) ) ) / 2 ) * 1 mm; if(( ( abs(trbl5 - trbl6) ) <> 1.2 ) or ( ( trbl5 - trbl6 ) <> 0 ); ( ( 3 - ( 2.40 * cos(30 deg) ) ) / 2 ) * 1 mm; 1 mm)))"
equation "tr6_left = if(( trbl5 < trbl6 ) and ( ( abs(trbl5 - trbl6) ) <> 1.2 ) and ( ( trbl5 - trbl6 ) <> 0 ); 3 mm - ( ( 3 mm - ( ( ( 2.4 * cos(30 deg) ) * 1 mm ) ) ) / 2 ) - ( ( ( trbl6 - trbl5 ) * 2 * cos(30 deg) ) * 1 mm ); if(( trbl5 > trbl6 ) and ( ( abs(trbl5 - trbl6) ) <> 1.2 ) and ( ( trbl5 - trbl6 ) <> 0 ); ( ( 3 - ( 2.40 * cos(30 deg) ) ) / 2 ) * 1 mm; if(( ( abs(trbl6 - trbl5) ) <> 1.2 ) or ( ( trbl5 - trbl6 ) <> 0 ); ( ( 3 - ( 2.40 * cos(30 deg) ) ) / 2 ) * 1 mm; 1 mm)))"
equation "tr6_right = if(( trbl6 > trbl7 ) and ( ( abs(trbl6 - trbl7) ) <> 1.2 ) and ( ( trbl6 - trbl7 ) <> 0 ); 3 mm - ( ( 3 mm - ( ( ( 2.4 * cos(30 deg) ) * 1 mm ) ) ) / 2 ) - ( ( ( trbl6 - trbl7 ) * 2 * cos(30 deg) ) * 1 mm ); if(( trbl6 < trbl7 ) and ( ( abs(trbl6 - trbl7) ) <> 1.2 ) and ( ( trbl6 - trbl7 ) <> 0 ); ( ( 3 - ( 2.40 * cos(30 deg) ) ) / 2 ) * 1 mm; if(( ( abs(trbl6 - trbl7) ) <> 1.2 ) or ( ( trbl6 - trbl7 ) <> 0 ); ( ( 3 - ( 2.40 * cos(30 deg) ) ) / 2 ) * 1 mm; 1 mm)))"
equation "tr7_left = if(( trbl6 < trbl7 ) and ( ( abs(trbl6 - trbl7) ) <> 1.2 ) and ( ( trbl6 - trbl7 ) <> 0 ); 3 mm - ( ( 3 mm - ( ( ( 2.4 * cos(30 deg) ) * 1 mm ) ) ) / 2 ) - ( ( ( trbl7 - trbl6 ) * 2 * cos(30 deg) ) * 1 mm ); if(( trbl6 > trbl7 ) and ( ( abs(trbl6 - trbl7) ) <> 1.2 ) and ( ( trbl6 - trbl7 ) <> 0 ); ( ( 3 - ( 2.40 * cos(30 deg) ) ) / 2 ) * 1 mm; if(( ( abs(trbl7 - trbl6) ) <> 1.2 ) or ( ( trbl6 - trbl7 ) <> 0 ); ( ( 3 - ( 2.40 * cos(30 deg) ) ) / 2 ) * 1 mm; 1 mm)))"
equation "tr7_right = if(( trbl7 > trbl8 ) and ( ( abs(trbl7 - trbl8) ) <> 1.2 ) and ( ( trbl7 - trbl8 ) <> 0 ); 3.5 mm - ( ( 3.5 mm - ( ( ( 2.4 * cos(30 deg) ) * 1 mm ) ) ) / 2 ) - ( ( ( trbl7 - trbl8 ) * 2 * cos(30 deg) ) * 1 mm ); if(( trbl7 < trbl8 ) and ( ( abs(trbl7 - trbl8) ) <> 1.2 ) and ( ( trbl7 - trbl8 ) <> 0 ); ( ( 3.5 - ( 2.40 * cos(30 deg) ) ) / 2 ) * 1 mm; if(( ( abs(trbl7 - trbl8) ) <> 1.2 ) or ( ( trbl7 - trbl8 ) <> 0 ); ( ( 3.5 - ( 2.40 * cos(30 deg) ) ) / 2 ) * 1 mm; 1 mm)))"
equation "tr8_left = if(( trbl7 < trbl8 ) and ( ( abs(trbl7 - trbl8) ) <> 1.2 ) and ( ( trbl7 - trbl8 ) <> 0 ); 3.5 mm - ( ( 3.5 mm - ( ( ( 2.4 * cos(30 deg) ) * 1 mm ) ) ) / 2 ) - ( ( ( trbl8 - trbl7 ) * 2 * cos(30 deg) ) * 1 mm ); if(( trbl7 > trbl8 ) and ( ( abs(trbl7 - trbl8) ) <> 1.2 ) and ( ( trbl7 - trbl8 ) <> 0 ); ( ( 3.5 - ( 2.40 * cos(30 deg) ) ) / 2 ) * 1 mm; if(( ( abs(trbl8 - trbl7) ) <> 1.2 ) or ( ( trbl7 - trbl8 ) <> 0 ); ( ( 3.5 - ( 2.40 * cos(30 deg) ) ) / 2 ) * 1 mm; 1 mm)))"
equation "tl_br1 = 1"
equation "tlbr1 = ( -0.025 * tl_br1 ^ 3 + 0.15 * tl_br1 ^ 2 - 0.625 * tl_br1 + 3 )"
equation "tl_br2 = 2"
equation "tlbr2 = ( -0.025 * tl_br2 ^ 3 + 0.15 * tl_br2 ^ 2 - 0.625 * tl_br2 + 3 )"
equation "tl_br3 = 3"
equation "tlbr3 = ( -0.025 * tl_br3 ^ 3 + 0.15 * tl_br3 ^ 2 - 0.625 * tl_br3 + 3 )"
equation "tl_br4 = 2"
equation "tlbr4 = ( -0.025 * tl_br4 ^ 3 + 0.15 * tl_br4 ^ 2 - 0.625 * tl_br4 + 3 )"
equation "tl_br5 = 0"
equation "tlbr5 = ( -0.025 * tl_br5 ^ 3 + 0.15 * tl_br5 ^ 2 - 0.625 * tl_br5 + 3 )"
equation "tl_br6 = 3"
equation "tlbr6 = ( -0.025 * tl_br6 ^ 3 + 0.15 * tl_br6 ^ 2 - 0.625 * tl_br6 + 3 )"
equation "tl_br7 = 2"
equation "tlbr7 = ( -0.025 * tl_br7 ^ 3 + 0.15 * tl_br7 ^ 2 - 0.625 * tl_br7 + 3 )"
equation "tl_br8 = 3"
equation "tlbr8 = ( -0.025 * tl_br8 ^ 3 + 0.15 * tl_br8 ^ 2 - 0.625 * tl_br8 + 3 )"
equation "tl1_left = if(( tlbr1 > tlbr2 ) and ( ( abs(tlbr1 - tlbr2) ) <> 1.2 ) and ( ( tlbr1 - tlbr2 ) <> 0 ); 3 mm - ( ( 3 mm - ( ( ( 2.4 * cos(30 deg) ) * 1 mm ) ) ) / 2 ) - ( ( ( tlbr1 - tlbr2 ) * 2 * cos(30 deg) ) * 1 mm ); if(( tlbr1 < tlbr2 ) and ( ( abs(tlbr1 - tlbr2) ) <> 1.2 ) and ( ( tlbr1 - tlbr2 ) <> 0 ); ( ( 3 - ( 2.40 * cos(30 deg) ) ) / 2 ) * 1 mm; if(( ( abs(tlbr1 - tlbr2) ) <> 1.2 ) or ( ( tlbr1 - tlbr2 ) <> 0 ); ( ( 3 - ( 2.40 * cos(30 deg) ) ) / 2 ) * 1 mm; 1 mm)))"
equation "tl2_right = if(( tlbr1 < tlbr2 ) and ( ( abs(tlbr1 - tlbr2) ) <> 1.2 ) and ( ( tlbr1 - tlbr2 ) <> 0 ); 3 mm - ( ( 3 mm - ( ( ( 2.4 * cos(30 deg) ) * 1 mm ) ) ) / 2 ) - ( ( ( tlbr2 - tlbr1 ) * 2 * cos(30 deg) ) * 1 mm ); if(( tlbr1 > tlbr2 ) and ( ( abs(tlbr1 - tlbr2) ) <> 1.2 ) and ( ( tlbr1 - tlbr2 ) <> 0 ); ( ( 3 - ( 2.40 * cos(30 deg) ) ) / 2 ) * 1 mm; if(( ( abs(tlbr2 - tlbr1) ) <> 1.2 ) or ( ( tlbr1 - tlbr2 ) <> 0 ); ( ( 3 - ( 2.40 * cos(30 deg) ) ) / 2 ) * 1 mm; 1 mm)))"
equation "tl2_left = if(( tlbr2 > tlbr3 ) and ( ( abs(tlbr2 - tlbr3) ) <> 1.2 ) and ( ( tlbr2 - tlbr3 ) <> 0 ); 3 mm - ( ( 3 mm - ( ( ( 2.4 * cos(30 deg) ) * 1 mm ) ) ) / 2 ) - ( ( ( tlbr2 - tlbr3 ) * 2 * cos(30 deg) ) * 1 mm ); if(( tlbr2 < tlbr3 ) and ( ( abs(tlbr2 - tlbr3) ) <> 1.2 ) and ( ( tlbr2 - tlbr3 ) <> 0 ); ( ( 3 - ( 2.40 * cos(30 deg) ) ) / 2 ) * 1 mm; if(( ( abs(tlbr2 - tlbr3) ) <> 1.2 ) or ( ( tlbr2 - tlbr3 ) <> 0 ); ( ( 3 - ( 2.40 * cos(30 deg) ) ) / 2 ) * 1 mm; 1 mm)))"
equation "tl3_right = if(( tlbr2 < tlbr3 ) and ( ( abs(tlbr2 - tlbr3) ) <> 1.2 ) and ( ( tlbr2 - tlbr3 ) <> 0 ); 3 mm - ( ( 3 mm - ( ( ( 2.4 * cos(30 deg) ) * 1 mm ) ) ) / 2 ) - ( ( ( tlbr3 - tlbr2 ) * 2 * cos(30 deg) ) * 1 mm ); if(( tlbr2 > tlbr3 ) and ( ( abs(tlbr2 - tlbr3) ) <> 1.2 ) and ( ( tlbr2 - tlbr3 ) <> 0 ); ( ( 3 - ( 2.40 * cos(30 deg) ) ) / 2 ) * 1 mm; if(( ( abs(tlbr3 - tlbr2) ) <> 1.2 ) or ( ( tlbr2 - tlbr3 ) <> 0 ); ( ( 3 - ( 2.40 * cos(30 deg) ) ) / 2 ) * 1 mm; 1 mm)))"
equation "tl3_left = if(( tlbr3 > tlbr4 ) and ( ( abs(tlbr3 - tlbr4) ) <> 1.2 ) and ( ( tlbr3 - tlbr4 ) <> 0 ); 3 mm - ( ( 3 mm - ( ( ( 2.4 * cos(30 deg) ) * 1 mm ) ) ) / 2 ) - ( ( ( tlbr3 - tlbr4 ) * 2 * cos(30 deg) ) * 1 mm ); if(( tlbr3 < tlbr4 ) and ( ( abs(tlbr3 - tlbr4) ) <> 1.2 ) and ( ( tlbr3 - tlbr4 ) <> 0 ); ( ( 3 - ( 2.40 * cos(30 deg) ) ) / 2 ) * 1 mm; if(( ( abs(tlbr3 - tlbr4) ) <> 1.2 ) or ( ( tlbr3 - tlbr4 ) <> 0 ); ( ( 3 - ( 2.40 * cos(30 deg) ) ) / 2 ) * 1 mm; 1 mm)))"
equation "tl4_right = if(( tlbr3 < tlbr4 ) and ( ( abs(tlbr3 - tlbr4) ) <> 1.2 ) and ( ( tlbr3 - tlbr4 ) <> 0 ); 3 mm - ( ( 3 mm - ( ( ( 2.4 * cos(30 deg) ) * 1 mm ) ) ) / 2 ) - ( ( ( tlbr4 - tlbr3 ) * 2 * cos(30 deg) ) * 1 mm ); if(( tlbr3 > tlbr4 ) and ( ( abs(tlbr3 - tlbr4) ) <> 1.2 ) and ( ( tlbr3 - tlbr4 ) <> 0 ); ( ( 3 - ( 2.40 * cos(30 deg) ) ) / 2 ) * 1 mm; if(( ( abs(tlbr4 - tlbr3) ) <> 1.2 ) or ( ( tlbr3 - tlbr4 ) <> 0 ); ( ( 3 - ( 2.40 * cos(30 deg) ) ) / 2 ) * 1 mm; 1 mm)))"
equation "tl4_left = if(( tlbr4 > tlbr5 ) and ( ( abs(tlbr4 - tlbr5) ) <> 1.2 ) and ( ( tlbr4 - tlbr5 ) <> 0 ); 3 mm - ( ( 3 mm - ( ( ( 2.4 * cos(30 deg) ) * 1 mm ) ) ) / 2 ) - ( ( ( tlbr4 - tlbr5 ) * 2 * cos(30 deg) ) * 1 mm ); if(( tlbr4 < tlbr5 ) and ( ( abs(tlbr4 - tlbr5) ) <> 1.2 ) and ( ( tlbr4 - tlbr5 ) <> 0 ); ( ( 3 - ( 2.40 * cos(30 deg) ) ) / 2 ) * 1 mm; if(( ( abs(tlbr4 - tlbr5) ) <> 1.2 ) or ( ( tlbr4 - tlbr5 ) <> 0 ); ( ( 3 - ( 2.40 * cos(30 deg) ) ) / 2 ) * 1 mm; 1 mm)))"
equation "tl5_right = if(( tlbr4 < tlbr5 ) and ( ( abs(tlbr4 - tlbr5) ) <> 1.2 ) and ( ( tlbr4 - tlbr5 ) <> 0 ); 3 mm - ( ( 3 mm - ( ( ( 2.4 * cos(30 deg) ) * 1 mm ) ) ) / 2 ) - ( ( ( tlbr5 - tlbr4 ) * 2 * cos(30 deg) ) * 1 mm ); if(( tlbr4 > tlbr5 ) and ( ( abs(tlbr4 - tlbr5) ) <> 1.2 ) and ( ( tlbr4 - tlbr5 ) <> 0 ); ( ( 3 - ( 2.40 * cos(30 deg) ) ) / 2 ) * 1 mm; if(( ( abs(tlbr5 - tlbr4) ) <> 1.2 ) or ( ( tlbr4 - tlbr5 ) <> 0 ); ( ( 3 - ( 2.40 * cos(30 deg) ) ) / 2 ) * 1 mm; 1 mm)))"
equation "tl5_left = if(( tlbr5 > tlbr6 ) and ( ( abs(tlbr5 - tlbr6) ) <> 1.2 ) and ( ( tlbr5 - tlbr6 ) <> 0 ); 3 mm - ( ( 3 mm - ( ( ( 2.4 * cos(30 deg) ) * 1 mm ) ) ) / 2 ) - ( ( ( tlbr5 - tlbr6 ) * 2 * cos(30 deg) ) * 1 mm ); if(( tlbr5 < tlbr6 ) and ( ( abs(tlbr5 - tlbr6) ) <> 1.2 ) and ( ( tlbr5 - tlbr6 ) <> 0 ); ( ( 3 - ( 2.40 * cos(30 deg) ) ) / 2 ) * 1 mm; if(( ( abs(tlbr5 - tlbr6) ) <> 1.2 ) or ( ( tlbr5 - tlbr6 ) <> 0 ); ( ( 3 - ( 2.40 * cos(30 deg) ) ) / 2 ) * 1 mm; 1 mm)))"
equation "tl6_right = if(( tlbr5 < tlbr6 ) and ( ( abs(tlbr5 - tlbr6) ) <> 1.2 ) and ( ( tlbr5 - tlbr6 ) <> 0 ); 3 mm - ( ( 3 mm - ( ( ( 2.4 * cos(30 deg) ) * 1 mm ) ) ) / 2 ) - ( ( ( tlbr6 - tlbr5 ) * 2 * cos(30 deg) ) * 1 mm ); if(( tlbr5 > tlbr6 ) and ( ( abs(tlbr5 - tlbr6) ) <> 1.2 ) and ( ( tlbr5 - tlbr6 ) <> 0 ); ( ( 3 - ( 2.40 * cos(30 deg) ) ) / 2 ) * 1 mm; if(( ( abs(tlbr6 - tlbr5) ) <> 1.2 ) or ( ( tlbr5 - tlbr6 ) <> 0 ); ( ( 3 - ( 2.40 * cos(30 deg) ) ) / 2 ) * 1 mm; 1 mm)))"
equation "tl6_left = if(( tlbr6 > tlbr7 ) and ( ( abs(tlbr6 - tlbr7) ) <> 1.2 ) and ( ( tlbr6 - tlbr7 ) <> 0 ); 3 mm - ( ( 3 mm - ( ( ( 2.4 * cos(30 deg) ) * 1 mm ) ) ) / 2 ) - ( ( ( tlbr6 - tlbr7 ) * 2 * cos(30 deg) ) * 1 mm ); if(( tlbr6 < tlbr7 ) and ( ( abs(tlbr6 - tlbr7) ) <> 1.2 ) and ( ( tlbr6 - tlbr7 ) <> 0 ); ( ( 3 - ( 2.40 * cos(30 deg) ) ) / 2 ) * 1 mm; if(( ( abs(tlbr6 - tlbr7) ) <> 1.2 ) or ( ( tlbr6 - tlbr7 ) <> 0 ); ( ( 3 - ( 2.40 * cos(30 deg) ) ) / 2 ) * 1 mm; 1 mm)))"
equation "tl7_right = if(( tlbr6 < tlbr7 ) and ( ( abs(tlbr6 - tlbr7) ) <> 1.2 ) and ( ( tlbr6 - tlbr7 ) <> 0 ); 3 mm - ( ( 3 mm - ( ( ( 2.4 * cos(30 deg) ) * 1 mm ) ) ) / 2 ) - ( ( ( tlbr7 - tlbr6 ) * 2 * cos(30 deg) ) * 1 mm ); if(( tlbr6 > tlbr7 ) and ( ( abs(tlbr6 - tlbr7) ) <> 1.2 ) and ( ( tlbr6 - tlbr7 ) <> 0 ); ( ( 3 - ( 2.40 * cos(30 deg) ) ) / 2 ) * 1 mm; if(( ( abs(tlbr7 - tlbr6) ) <> 1.2 ) or ( ( tlbr6 - tlbr7 ) <> 0 ); ( ( 3 - ( 2.40 * cos(30 deg) ) ) / 2 ) * 1 mm; 1 mm)))"
equation "tl7_left = if(( tlbr7 > tlbr8 ) and ( ( abs(tlbr7 - tlbr8) ) <> 1.2 ) and ( ( tlbr7 - tlbr8 ) <> 0 ); 3.5 mm - ( ( 3.5 mm - ( ( ( 2.4 * cos(30 deg) ) * 1 mm ) ) ) / 2 ) - ( ( ( tlbr7 - tlbr8 ) * 2 * cos(30 deg) ) * 1 mm ); if(( tlbr7 < tlbr8 ) and ( ( abs(tlbr7 - tlbr8) ) <> 1.2 ) and ( ( tlbr7 - tlbr8 ) <> 0 ); ( ( 3.5 - ( 2.40 * cos(30 deg) ) ) / 2 ) * 1 mm; if(( ( abs(tlbr7 - tlbr8) ) <> 1.2 ) or ( ( tlbr7 - tlbr8 ) <> 0 ); ( ( 3.5 - ( 2.40 * cos(30 deg) ) ) / 2 ) * 1 mm; 1 mm)))"
equation "tl8_right = if(( tlbr7 < tlbr8 ) and ( ( abs(tlbr7 - tlbr8) ) <> 1.2 ) and ( ( tlbr7 - tlbr8 ) <> 0 ); 3.5 mm - ( ( 3.5 mm - ( ( ( 2.4 * cos(30 deg) ) * 1 mm ) ) ) / 2 ) - ( ( ( tlbr8 - tlbr7 ) * 2 * cos(30 deg) ) * 1 mm ); if(( tlbr7 > tlbr8 ) and ( ( abs(tlbr7 - tlbr8) ) <> 1.2 ) and ( ( tlbr7 - tlbr8 ) <> 0 ); ( ( 3.5 - ( 2.40 * cos(30 deg) ) ) / 2 ) * 1 mm; if(( ( abs(tlbr8 - tlbr7) ) <> 1.2 ) or ( ( tlbr7 - tlbr8 ) <> 0 ); ( ( 3.5 - ( 2.40 * cos(30 deg) ) ) / 2 ) * 1 mm; 1 mm)))"
equation "d61 = ( 2.3 / 2 ) * 1 mm"
equation "d62 = ( 8.6 / 2 ) * 1 mm"
equation "d63 = d61 * 2"
equation "d64 = d62 * 2"
equation "d65 = -32.35 mm"
equation "d67 = -d65"
equation "d68 = ( 2.5 * 0.5 ) * 1 mm"
equation "d70 = ( ( ( 4.3 - 1.25 ) / sin(45 deg) ) * 1 mm )"
equation "d71 = d68"
equation "d72 = d68"
equation "d73 = ( 1 * 0.5 ) * 1 mm"
equation "d74 = ( 1 * 0.5 ) * 1 mm"
equation "d75 = d74"
equation "d76 = d73"
equation "d77 = d65"
equation "d83 = 32.5 deg"
equation "d84 = -d83"
equation "half_cut = ( ( 3 - ( 2.40 * cos(30 deg) ) ) / 2 ) * 1 mm"
equation "d87 = ( 1 / 2 ) * 1 mm"
equation "d88 = trbl1 * mm"
equation "d90 = trbl2 * mm"
equation "d91 = d89"
equation "d92 = trbl3 * mm"
equation "d93 = d89"
equation "d94 = trbl4 * mm"
equation "d95 = d89"
equation "d96 = trbl5 * mm"
equation "d97 = d89"
equation "d98 = trbl6 * mm"
equation "d99 = d89"
equation "d100 = trbl7 * mm"
equation "d102 = trbl8 * mm"
equation "d105 = half_cut"
equation "d108 = if(( 3 > trbl1 ) and ( ( abs(3 - trbl1) ) <> 1.2 ) and ( ( 3 - trbl1 ) <> 0 ); 3 mm - ( ( 3 mm - ( ( ( 2.4 * cos(30 deg) ) * 1 mm ) ) ) / 2 ) - ( ( ( 3 - trbl1 ) * 2 * cos(30 deg) ) * 1 mm ); if(( 3 < trbl1 ) and ( ( abs(3 - trbl1) ) <> 1.2 ) and ( ( 3 - trbl1 ) <> 0 ); ( ( 3 - ( 2.40 * cos(30 deg) ) ) / 2 ) * 1 mm; if(( ( abs(3 - trbl1) ) <> 1.2 ) or ( ( 3 - trbl1 ) <> 0 ); ( ( 3 - ( 2.40 * cos(30 deg) ) ) / 2 ) * 1 mm; 1 mm)))"
equation "d109 = tr1_right"
equation "d110 = tr2_left"
equation "d111 = tr2_right"
equation "d112 = tr3_left"
equation "d113 = tr3_right"
equation "d114 = tr4_left"
equation "d115 = tr4_right"
equation "d116 = tr5_left"
equation "d117 = tr5_right"
equation "d118 = tr6_left"
equation "d119 = tr6_right"
equation "d120 = tr7_left"
equation "d121 = tr7_right"
equation "d122 = tr8_left"
equation "d123 = 180 deg - d83"
equation "d124 = trbl8 * mm"
equation "d127 = d126"
equation "d128 = d124"
equation "d129 = d126"
equation "d130 = d126"
equation "d131 = d86"
equation "d132 = d87"
equation "d133 = tlbr1 * mm"
equation "d134 = d89"
equation "d135 = tlbr2 * mm"
equation "d136 = d89"
equation "d137 = tlbr3 * mm"
equation "d138 = d89"
equation "d139 = tlbr4 * mm"
equation "d140 = d89"
equation "d141 = tlbr5 * mm"
equation "d142 = d89"
equation "d143 = tlbr6 * mm"
equation "d144 = d89"
equation "d145 = tlbr7 * mm"
equation "d146 = d101"
equation "d147 = tlbr8 * mm"
equation "d148 = d103"
equation "d149 = d104"
equation "d150 = d89"
equation "d152 = half_cut"
equation "d153 = if(( 3 > tlbr1 ) and ( ( abs(3 - tlbr1) ) <> 1.2 ) and ( ( 3 - tlbr1 ) <> 0 ); 3 mm - ( ( 3 mm - ( ( ( 2.4 * cos(30 deg) ) * 1 mm ) ) ) / 2 ) - ( ( ( 3 - tlbr1 ) * 2 * cos(30 deg) ) * 1 mm ); if(( 3 < tlbr1 ) and ( ( abs(3 - tlbr1) ) <> 1.2 ) and ( ( 3 - tlbr1 ) <> 0 ); ( ( 3 - ( 2.40 * cos(30 deg) ) ) / 2 ) * 1 mm; if(( ( abs(3 - tlbr1) ) <> 1.2 ) or ( ( 3 - tlbr1 ) <> 0 ); ( ( 3 - ( 2.40 * cos(30 deg) ) ) / 2 ) * 1 mm; 1 mm)))"
equation "d154 = tl1_left"
equation "d155 = tl2_right"
equation "d156 = tl2_left"
equation "d157 = tl3_right"
equation "d158 = tl3_left"
equation "d159 = tl4_right"
equation "d160 = tl4_left"
equation "d161 = tl5_right"
equation "d162 = tl5_left"
equation "d163 = tl6_right"
equation "d164 = tl6_left"
equation "d165 = tl7_right"
equation "d166 = tl7_left"
equation "d167 = tl8_right"
equation "d168 = tlbr8 * mm"
equation "d169 = d83"
equation "d170 = d126"
equation "d171 = d126"
equation "d172 = d168"
equation "d173 = d126"
equation "d174 = d126"
